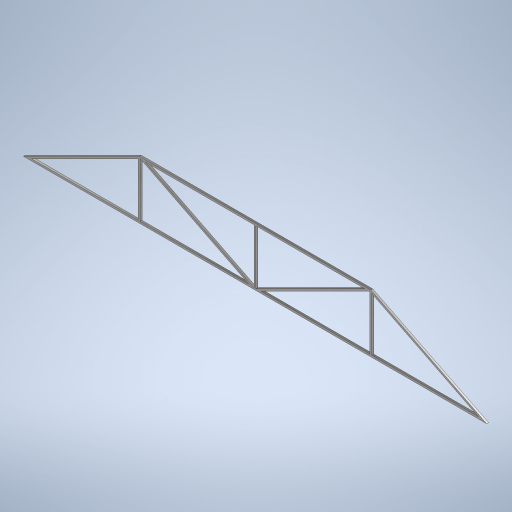
# Autodesk Inventor part: Truss
Saved by Autodesk Inventor 2023 (Build 270158000, 158)
## iProperties
Created: 2023-11-29
Part Number: Truss
Material: Stainless Steel
Document SubType Name: Modeling
Designer: Gage
Density: 8 g/cm^3
Appearance: Semi-Polished
Author: Gage
Autodesk Inventor part; units mm, degrees
ref_plane "YZ Plane" through (0, 0, 0) normal (1, 0, 0) x (0, 1, 0)
ref_plane "XZ Plane" through (0, 0, 0) normal (0, 1, 0) x (-1, 0, 0)
ref_plane "XY Plane" through (0, 0, 0) normal (0, 0, 1) x (1, 0, 0)
sketch "Sketch1" plane through (0, 0, 0) normal (0, 0, 1) x (1, 0, 0)
  line L0 (0, 0) -> (609.6, 0)
  line L1 (152.4, 0) -> (152.4, 76.2)
  line L2 (152.4, 0) -> (228.6, 0) construction
  line L3 (304.8, 0) -> (304.8, 76.2)
  line L4 (457.2, 0) -> (457.2, 76.2)
  line L5 (457.2, 76.2) -> (609.6, 0)
  line L6 (457.2, 76.2) -> (304.8, 76.2)
  line L7 (152.4, 76.2) -> (0, 0)
  line L8 (152.4, 76.2) -> (304.8, 76.2)
  line L9 (304.8, 0) -> (457.2, 76.2)
  line L10 (304.8, 0) -> (152.4, 76.2)
  line L11 (151.13, 2.54) -> (151.13, 72.7252)
  line L12 (10.7596, 2.54) -> (151.13, 72.7252)
  line L13 (10.7596, 2.54) -> (151.13, 2.54)
  line L14 (458.47, 2.54) -> (458.47, 72.7252)
  line L15 (598.8404, 2.54) -> (458.47, 72.7252)
  line L16 (598.8404, 2.54) -> (458.47, 2.54)
  line L17 (153.67, 2.54) -> (153.67, 74.1451)
  line L18 (151.13, 2.54) -> (296.8802, 2.54)
  line L19 (299.1204, 0) -> (299.3101, -0.0949)
  line L20 (153.67, 74.1451) -> (296.8802, 2.54)
  line L21 (455.93, 2.54) -> (455.93, 74.1451)
  line L22 (458.47, 2.54) -> (312.7198, 2.54)
  line L23 (455.93, 74.1451) -> (312.7198, 2.54)
  line L24 (160.3198, 73.66) -> (303.53, 73.66)
  line L25 (303.53, 73.66) -> (303.53, 2.0549)
  line L26 (160.3198, 73.66) -> (303.53, 2.0549)
  line L27 (449.2802, 73.66) -> (306.07, 73.66)
  line L28 (306.07, 73.66) -> (306.07, 2.0549)
  line L29 (449.2802, 73.66) -> (306.07, 2.0549)
  point P0 (149.86, 73.66)
  point P1 (160.3375, 73.66)
  point P2 (449.2625, 73.66)
  dimension "d0" = 609.6
  dimension "d1" = 152.4
  dimension "d2" = 152.4
  dimension "d3" = 152.4
  dimension "d4" = 76.2
  dimension "d5" = 90
  dimension "d7" = 1.27
  dimension "d10" = 1.27
  dimension "d12" = 2.54
  dimension "d13" = 1.27
  dimension "d15" = 1.27
  dimension "d16" = 90
  dimension "d17" = 2.54
  dimension "d18" = 2.54
  dimension "d19" = 1.27
  constraints: 60 end point, 10 symmetric about line, 7 point on line, 5 parallel, 5 vertical, 3 horizontal, 2 midpoint, 2 perpendicular, 1 collinear
  measures "d0" distance of L0.start L0.end
  measures "d1" distance of L0.start L1.start
  measures "d2" distance of L1.start point (304.8, 0)
  measures "d3" distance of L3.start L4.start
  measures "d4" distance of L1.start L1.end
  measures "d5" angle of L2 L1
  measures "d7" distance from line of L1 L11.start
  measures "d10" distance between parallel lines of L1 L17
  measures "d12" distance between parallel lines of L8 L24
  measures "d13" distance between parallel lines of L3 L25
  measures "d15" distance between parallel lines of L10 L20
  measures "d16" angle of L17 L18
  measures "d17" distance between parallel lines of L0 L13
  measures "d18" distance between parallel lines of L7 L12
  measures "d19" distance between parallel lines of L26 L10
extrude "Extrusion1" add sketch "Sketch1" along normal blind 2.54
body "Solid1"
